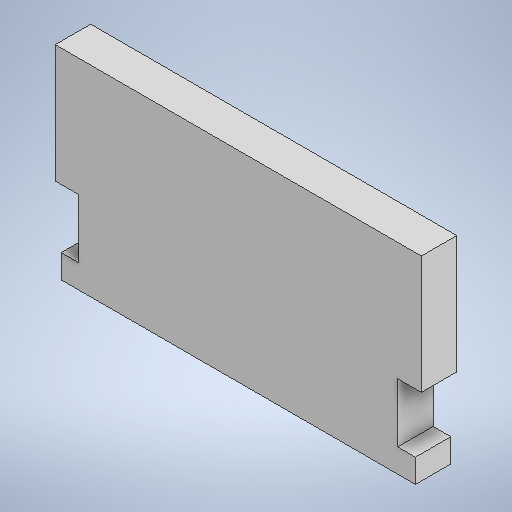
# Autodesk Inventor part: Piston_FloorHinge02
Saved by Autodesk Inventor 2025.2 (Build 292293000, 293)
## iProperties
Created: 2025-04-08
Part Number: Piston_FloorHinge02
Material: Generic
Document SubType Name: Sheet Metal
Designer: Victor
Density: 1 g/cm^3
Sheet Metal Rule: Default_mm
Appearance: Default
Flat Pattern Width: 1.7 cm
Flat Pattern Length: 3.1 cm
Flat Pattern Area: 5.27 cm^2
Sheet Metal Width: 17,000 mm
Sheet Metal Length: 31,000 mm
Sheet Metal Area: 527,000 mm^2
Author: Victor
Autodesk Inventor part; units mm, degrees
ref_plane "YZ Plane" through (0, 0, 0) normal (1, 0, 0) x (0, 1, 0)
ref_plane "XZ Plane" through (0, 0, 0) normal (0, 1, 0) x (-1, 0, 0)
ref_plane "XY Plane" through (0, 0, 0) normal (0, 0, 1) x (1, 0, 0)
sketch "Sketch1" plane through (0, 0, 0) normal (0, 0, 1) x (1, 0, 0)
  line L0 (-11.7274, -1.8139) -> (15.2726, -1.8139)
  line L1 (15.2726, -1.8139) -> (15.2726, 13.1861)
  line L2 (15.2726, 13.1861) -> (-11.7274, 13.1861)
  line L3 (-11.7274, 13.1861) -> (-11.7274, -1.8139)
  line L4 (-13.2274, -1.8139) -> (16.7726, -1.8139)
  line L5 (16.7726, -1.8139) -> (16.7726, -3.8139)
  line L6 (16.7726, -3.8139) -> (-13.2274, -3.8139)
  line L7 (-13.2274, -3.8139) -> (-13.2274, -1.8139)
  line L8 (-11.7274, 3.1861) -> (-13.7274, 3.1861)
  line L9 (-13.7274, 3.1861) -> (-13.7274, 13.1861)
  line L10 (-13.7274, 13.1861) -> (-11.7274, 13.1861)
  line L11 (-11.7274, 13.1861) -> (-11.7274, 3.1861)
  line L12 (1.7726, 13.1861) -> (1.7726, -1.8139)
  line L13 (17.2726, 13.1861) -> (15.2726, 13.1861)
  line L14 (17.2726, 3.1861) -> (17.2726, 13.1861)
  line L15 (15.2726, 3.1861) -> (17.2726, 3.1861)
  point P0 (0, 0)
  dimension "d0" = 27
  dimension "d1" = 30
  dimension "d2" = 2
  dimension "d3" = 15
  dimension "d4" = 2
  dimension "d5" = 10
  dimension "d6" = 5
  measures "d0" distance of L2.end L2.start
  measures "d1" distance of L6.start L6.end
  measures "d2" distance of L4.end L6.start
  measures "d3" distance between parallel lines of L2 L0
  measures "d4" distance of L10.start L11.start
  measures "d5" distance of L9.start L10.start
  measures "d6" distance between parallel lines of L0 L8
extrude "Plate1" add sketch "Sketch1" along normal blind 3
equation "\"d0\" = L_Piston_Bottom + 2 * A_joint_tolerance"
equation "\"d2\" = d7"
equation "\"d4\" = d7"
equation "\"d10\" = Thickness"
equation "\"Thickness\" = plate_thickness"
equation "\"BendRadius\" = Thickness"
equation "\"BendReliefWidth\" = Thickness"
equation "\"BendReliefDepth\" = 0.5 * Thickness"
equation "\"CornerReliefSize\" = 4 * Thickness"
equation "\"MinimumRemnant\" = 2 * Thickness"
equation "\"TransitionRadius\" = BendRadius"
equation "\"JacobiRadiusSize\" = BendRadius"
equation "\"GapSize\" = Thickness"
equation "\"A_width\" = 46"
equation "\"A_joint_diameter\" = 16"
equation "\"A_joint_tolerance\" = 3"
equation "\"l___________\" = 0"
equation "\"l__________\" = 0"
equation "\"l_________\" = 0"
equation "\"rivet_diameter\" = 3.35"
equation "\"plate_thickness\" = 3"
equation "\"l________\" = 0"
equation "\"L_Piston_Top\" = 25"
equation "\"L_Piston_Bottom\" = 21"
equation "\"A_B_spacing\" = 2"
equation "\"thin_plate\" = 1.5"
equation "\"d7\" = 2"
body "Solid1"
